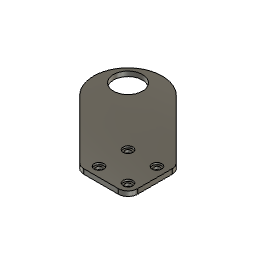
_Grip arm bracket front side.1cbf9639-d063-4f21-8cd9-8bfc683fe057 (Autodesk Fusion 360 design; units mm, degrees)
Autodesk Fusion 360 part; units mm, degrees
sketch "Sketch1" plane through (0, 0, 0) normal (0, 0, 1) x (1, 0, 0)
  line L0 (0, 0) -> (50, 0)
  line L1 (50, 0) -> (50, 50)
  line L2 (50, 50) -> (0, 50)
  line L3 (0, 50) -> (0, 0)
  dimension "d1" = 50
  dimension "d2" = 50
  constraint horizontal L0
  constraint vertical L1
  constraint horizontal L2
  constraint vertical L3
  constraint coincident L0.start L3.end
  measures "d1" distance of L0.start L0.end
  measures "d2" distance of L0.start L2.end
extrude "Extrude1" add sketch "Sketch1" along normal blind 5
sketch "Sketch2" plane through (0, 0, 0) normal (0, 0, 1) x (1, 0, 0)
  line L0 (0, 0) -> (50, 50)
  line L1 (50, 50) -> (-38.3883, 138.3883)
  line L2 (-38.3883, 138.3883) -> (-88.3883, 88.3883)
  line L3 (-88.3883, 88.3883) -> (0, 0)
  dimension "d5" = 125
  constraint perpendicular L0 L1
  constraint parallel L0 L2
  constraint parallel L1 L3
  constraint coincident L0.start L3.end
  measures "d5" distance of L0.start L2.end
extrude "Extrude2" add sketch "Sketch2" along normal blind 5
sketch "Sketch3" plane through (0, 0, 5) normal (0, 0, 1) x (-1, 0, 0)
  line L0 (0, 0) -> (-50, 0)
  line L1 (-50, 0) -> (-50, -50)
  line L2 (-50, -50) -> (38.3883, -138.3883)
  line L3 (38.3883, -138.3883) -> (88.3883, -88.3883)
  line L4 (88.3883, -88.3883) -> (0, 0)
  circle A0 centre (-10, -10) radius 5
  circle A1 centre (-40, -10) radius 5
  circle A2 centre (-40, -40) radius 5
  circle A3 centre (-10, -40) radius 5
  dimension "d8" = 10
  dimension "d9" = 10
  dimension "d10" = 10
  dimension "d11" = 10
  measures "d8" diameter of A0
  measures "d9" diameter of A1
  measures "d10" diameter of A2
  measures "d11" diameter of A3
extrude "Extrude3" cut sketch "Sketch3" against normal blind 2 contours A0 | A1 | A2 | A3
sketch "Sketch4" plane through (0, 0, 3) normal (0, 0, 1) x (-1, 0, 0)
  circle A0 centre (-10, -40) radius 5
  circle A1 centre (-10, -40) radius 3
  circle A2 centre (-40, -40) radius 3
  circle A3 centre (-10, -10) radius 3
  circle A4 centre (-40, -10) radius 3
  dimension "d14" = 6
  dimension "d15" = 6
  dimension "d16" = 6
  dimension "d17" = 6
  constraint concentric A0 A1
  measures "d14" diameter of A1
  measures "d15" diameter of A2
  measures "d16" diameter of A3
  measures "d17" diameter of A4
extrude "Extrude4" cut sketch "Sketch4" against normal blind 5 contours A1 | A2 | A3 | A4
sketch "Sketch5" plane through (0, 0, 5) normal (0, 0, 1) x (-1, 0, 0)
  circle A0 centre (-40, -40) radius 5
  circle A1 centre (-40, -10) radius 5
  circle A2 centre (-10, -40) radius 5
  circle A3 centre (-10, -10) radius 5
  line L0 (0, 0) -> (-50, 0)
  line L1 (-50, 0) -> (-50, -50)
  line L2 (-50, -50) -> (38.3883, -138.3883)
  line L3 (38.3883, -138.3883) -> (88.3883, -88.3883)
  line L4 (88.3883, -88.3883) -> (0, 0)
  circle A4 centre (50, -100) radius 15
  dimension "d20" = 30
  measures "d20" diameter of A4
extrude "Extrude5" cut sketch "Sketch5" against normal blind 5 contours A4
fillet "Fillet1" radius 35 2 edges at (-88.3883, 88.3883, 2.5) (-38.3883, 138.3883, 2.5)
fillet "Fillet2" radius 10 3 edges at (0, 0, 2.5) (50, 0, 2.5) (50, 50, 2.5)
